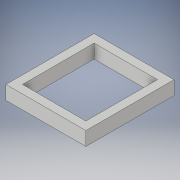
# Autodesk Inventor part: sop
Saved by Autodesk Inventor 2019 (Build 230136000, 136)
## iProperties
Created: 2022-02-05
Part Number: sop
Material: Generic
Document SubType Name: Modeling
Designer: josec
Density: 1 g/cm^3
Appearance: Default
Author: josec
Autodesk Inventor part; units mm, degrees
ref_plane "YZ Plane" through (0, 0, 0) normal (1, 0, 0) x (0, 1, 0)
ref_plane "XZ Plane" through (0, 0, 0) normal (0, 1, 0) x (-1, 0, 0)
ref_plane "XY Plane" through (0, 0, 0) normal (0, 0, 1) x (1, 0, 0)
sketch "Sketch1" plane through (0, 0, 0) normal (0, 1, 0) x (-1, 0, 0)
  line L0 (0, 0) -> (-29, 0)
  line L1 (-29, 0) -> (-29, -32)
  line L2 (-29, -32) -> (0, -32)
  line L3 (0, -32) -> (0, 0)
  dimension "d0" = 29
  dimension "d1" = 32
  constraints: 8 end point, 2 parallel, 1 horizontal, 1 perpendicular
  measures "d0" distance of L2.end L1.end
  measures "d1" distance of L1.end L0.end
extrude "Extrusion1" add sketch "Sketch1" along normal blind 5
sketch "Sketch3" plane through (0, 5, 0) normal (0, 1, 0) x (1, 0, 0)
  line L0 (29, 0) -> (29, 32) construction
  line L1 (0, 0) -> (29, 0) construction
  line L2 (29, 32) -> (0, 0) construction
  line L3 (3, 3) -> (26, 3)
  line L4 (26, 3) -> (26, 29)
  line L5 (26, 29) -> (3, 29)
  line L6 (3, 29) -> (3, 3)
  line L7 (3, 3) -> (26, 29) construction
  line L8 (26, 3) -> (3, 29) construction
  point P0 (14.5, 16)
  dimension "d4" = 23
  dimension "d5" = 26
  constraints: 14 end point, 3 midpoint, 2 parallel, 1 horizontal, 1 perpendicular
  measures "d4" distance of L5.end L4.end
  measures "d5" distance of L4.end L3.end
extrude "Extrusion2" cut sketch "Sketch3" against normal through all
body "Solid1"
